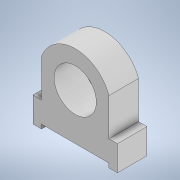
# Autodesk Inventor part: Assignment 2.5 - Guide Silder
Saved by Autodesk Inventor 2022 (Build 260153000, 153)
## iProperties
Created: 2021-05-23
Part Number: Assignment 2.5 - Guide Silder
Material: Generic
Document SubType Name: Modeling
Designer: Aaron
Density: 1 g/cm^3
Appearance: Default
Author: Aaron
Autodesk Inventor part; units mm, degrees
ref_plane "YZ Plane" through (0, 0, 0) normal (1, 0, 0) x (0, 1, 0)
ref_plane "XZ Plane" through (0, 0, 0) normal (0, 1, 0) x (-1, 0, 0)
ref_plane "XY Plane" through (0, 0, 0) normal (0, 0, 1) x (1, 0, 0)
sketch "Sketch1" plane through (0, 0, 0) normal (0, 0, 1) x (1, 0, 0)
  line L0 (0, 0) -> (12.7, 0)
  line L1 (12.7, 0) -> (12.7, 6.35)
  line L2 (12.7, 6.35) -> (114.3, 6.35)
  line L3 (114.3, 6.35) -> (114.3, 0)
  line L4 (114.3, 0) -> (127, 0)
  line L5 (127, 0) -> (127, 38.1)
  line L6 (127, 38.1) -> (114.3, 38.1)
  line L7 (0, 38.1) -> (12.7, 38.1)
  line L8 (0, 0) -> (0, 76.2)
  line L9 (0, 76.2) -> (63.5, 76.2)
  circle A0 centre (63.5, 76.2) radius 31.75
  arc A1 (114.3, 94.439) -> (12.7, 94.439) centre (63.5, 76.2) ccw
  line L10 (12.7, 38.1) -> (12.7, 94.439)
  line L11 (114.3, 38.1) -> (114.3, 94.439)
  dimension "d0" = 12.7
  dimension "d1" = 6.35
  dimension "d2" = 101.6
  dimension "d3" = 6.35
  dimension "d4" = 12.7
  dimension "d5" = 38.1
  dimension "d6" = 12.7
  dimension "d7" = 38.1
  dimension "d8" = 12.7
  dimension "d9" = 76.2
  dimension "d10" = 63.5
  dimension "d11" = 63.5
  dimension "d12" = 107.95
  constraints: 24 end point, 5 perpendicular, 3 vertical, 2 centre point, 2 coincident, 2 point on circle, 1 horizontal, 1 parallel, 1 point on line
  measures "d0" distance of L0.start L0.end
  measures "d1" distance of L0.end L1.end
  measures "d2" distance of L1.end L2.end
  measures "d3" distance of L2.end L3.end
  measures "d4" distance of L3.end L4.end
  measures "d5" distance of L4.end L5.end
  measures "d6" distance of L5.end L6.end
  measures "d7" distance of L0.start L7.start
  measures "d8" distance of L7.start L7.end
  measures "d9" distance of L0.start L8.end
  measures "d10" distance of L8.end L9.end
  measures "d11" diameter of A0
  measures "d12" diameter of A1
extrude "Extrusion1" add sketch "Sketch1" along normal blind 44.45 contours L8 L7 L10 A1 L11 L6 L5 L4 L3 L2 L1 L0
body "Solid1"
